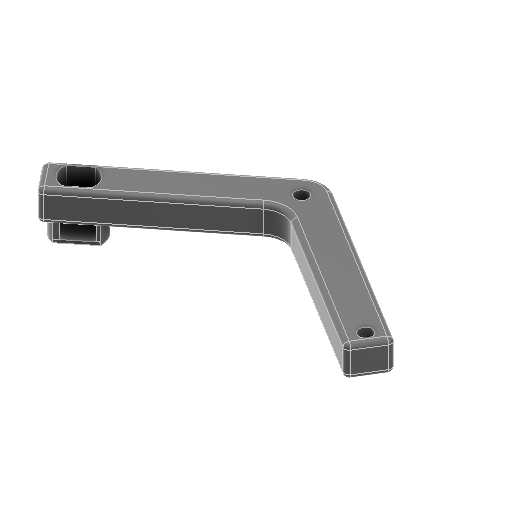
# Autodesk Inventor part: bogie
Saved by Autodesk Inventor 2025 (Build 290162010, 162A)
## iProperties
Created: 2024-08-06
Part Number: bogie
Material: Generic
Document SubType Name: Modeling
Designer: Pauline Simonnet
Density: 1 g/cm^3
Appearance: Smooth - Black
Author: Pauline Simonnet
Autodesk Inventor part; units mm, degrees
ref_plane "YZ Plane" through (0, 0, 0) normal (1, 0, 0) x (0, 1, 0)
ref_plane "XZ Plane" through (0, 0, 0) normal (0, 1, 0) x (-1, 0, 0)
ref_plane "XY Plane" through (0, 0, 0) normal (0, 0, 1) x (1, 0, 0)
sketch "Sketch1" plane through (0, 0, 0) normal (0, 1, 0) x (-1, 0, 0)
  line L0 (-464.4468, -188.2824) -> (-373.9516, -116.1994)
  line L1 (-373.9516, -116.1994) -> (-464.4468, -188.2824)
  line L2 (-464.4468, -188.2824) -> (-563.1339, -127.8985)
  line L3 (-563.1339, -127.8985) -> (-575.66, -148.3704)
  line L4 (-575.66, -148.3704) -> (-462.6384, -217.5251)
  line L5 (-373.9516, -116.1994) -> (-358.9986, -134.9719)
  line L6 (-358.9986, -134.9719) -> (-462.6384, -217.5251)
  line L7 (-462.6384, -217.5251) -> (-451.0106, -198.5213) construction
  line L8 (-462.6384, -217.5251) -> (-476.0378, -200.7031) construction
  circle A0 centre (-463.7684, -199.2538) radius 4.2
  circle A1 centre (-562.573, -142.3098) radius 4.3
  line L9 (-369.8895, -139.0445) -> (-380.7523, -147.6971)
  line L10 (-379.9517, -126.4122) -> (-390.8145, -135.0648)
  line L11 (-375.3209, -143.3708) -> (-385.3831, -130.7385) construction
  line L12 (-366.4751, -125.5857) -> (-380.352, -137.0546) construction
  arc A2 (-369.8895, -139.0445) -> (-379.9517, -126.4122) centre (-380.352, -137.0546) ccw
  arc A3 (-390.8145, -135.0648) -> (-380.7523, -147.6971) centre (-380.352, -137.0546) ccw
  point P0 (0, 0)
  dimension "d17" = 110
  dimension "d18" = 24
  dimension "d19" = 24
  dimension "d20" = 90
  dimension "d21" = 90
  dimension "d23" = 8.6
  dimension "d24" = 8.4
  dimension "d25" = 8
  dimension "d26" = 12
  dimension "d29" = 10.5
  dimension "d30" = 10.5
  dimension "d31" = 122
  dimension "d32" = 122
  dimension "d43" = 16.15
  dimension "d46" = 10.65
  dimension "d47" = 18
  constraints: 26 end point, 4 centre point, 4 midpoint, 4 point on circle, 1 coincident, 1 collinear, 1 perpendicular
  measures "d17" angle of L2 L0
  measures "d18" distance between parallel lines of L4 L2
  measures "d19" distance between parallel lines of L0 L6
  measures "d20" angle of L8 L6
  measures "d21" angle of L4 L7
  measures "d23" diameter of A1
  measures "d24" diameter of A0
  measures "d25" distance from line of L3 A1.centre
  measures "d26" distance from line of A1.centre L2
  measures "d29" distance from line of A0.centre L7
  measures "d30" distance from line of L8 A0.centre
  measures "d31" distance from line of L3 A0.centre
  measures "d32" distance from line of A0.centre L5
  measures "d43" distance between parallel lines of L10 L9
  measures "d46" radius of A3
  measures "d47" distance between parallel lines of L11 L5
extrude "Extrusion1" add sketch "Sketch1" along normal blind 20
fillet "Fillet1" radius 15 1 edges at (464.4468, 10, -188.2824)
fillet "Fillet2" radius 15 1 edges at (462.6384, 10, -217.5251)
fillet "Fillet3" radius 3 2 edges at (518.2699, 20, -155.3496) (415.0915, 20, -148.9689)
fillet "Fillet4" radius 3 3 edges at (462.8428, 20, -214.2198) (523.6288, 20, -180.2068) (406.7108, 20, -172.9766)
fillet "Fillet5" radius 3 3 edges at (462.8428, 0, -214.2198) (523.6288, 0, -180.2068) (406.7108, 0, -172.9766)
fillet "Fillet6" radius 3 2 edges at (518.2699, 0, -155.3496) (415.0915, 0, -148.9689)
fillet "Fillet7" radius 3 8 edges at (575.2014, 19.1213, -147.6209) (569.3969, 20, -138.1345) (563.5925, 19.1213, -128.6481) (563.1339, 10, -127.8985) (563.5925, 0.8787, -128.6481) (569.3969, 0, -138.1345) (575.2014, 0.8787, -147.6209) (575.66, 10, -148.3704)
fillet "Fillet8" radius 3 8 edges at (373.4042, 0.8787, -116.8867) (373.9516, 10, -116.1994) (373.4042, 19.1213, -116.8867) (366.4751, 20, -125.5857) (359.5461, 19.1213, -134.2846) (358.9986, 10, -134.9719) (359.5461, 0.8787, -134.2846) (366.4751, 0, -125.5857)
sketch "Sketch4" plane through (0, 0, 0) normal (0, -1, 0) x (1, 0, 0)
  arc A0 (379.9517, -126.4122) -> (369.8895, -139.0445) centre (380.352, -137.0546) ccw projected
  line L0 (368.3625, -139.1066) -> (381.7905, -149.8025)
  line L1 (369.8895, -139.0445) -> (380.7523, -147.6971) projected
  line L2 (365.9508, -139.7425) -> (380.5842, -151.3986)
  line L3 (394.6978, -137.0546) -> (377.3241, -122.7211)
  line L4 (454.3623, -184.0851) -> (374.4291, -120.4151) projected
  arc A1 (377.3241, -122.7211) -> (365.9508, -139.7425) centre (380.352, -137.0546) ccw
  arc A2 (380.5842, -151.3986) -> (394.6891, -136.553) centre (380.352, -137.0546) ccw
  arc A3 (380.0527, -124.8945) -> (368.3625, -139.1066) centre (380.352, -137.0546) ccw
  arc A4 (381.7905, -149.8025) -> (393.0533, -135.25) centre (380.352, -137.0546) ccw
  point P0 (0, 0)
  point P1 (379.9617, -124.8971)
  point P2 (393.1141, -135.748)
  dimension "d60" = 0
  dimension "d61" = 0
  dimension "d64" = 1
  dimension "d65" = 2
  constraints: 9 point on circle, 6 end point, 4 centre point, 4 point on line, 1 coincident, 1 parallel
  measures "d60" distance of A0.centre A3.centre
  measures "d61" distance of A0.centre A3.centre
  measures "d64" distance between parallel lines of L1 L0
  measures "d65" distance between parallel lines of L0 L2
extrude "Extrusion4" add sketch "Sketch4" along normal blind 10 contours L0 A4 L3 A2 L2 A1 A3
sketch "Sketch5" plane through (0, -10, 0) normal (0, -1, 0) x (1, 0, 0)
  arc A0 (383.8842, -150.9588) -> (394.6978, -137.0546) centre (380.352, -137.0546) ccw projected
  line L0 (394.6978, -137.0546) -> (377.413, -123.1311)
  arc A1 (380.5842, -151.3986) -> (394.6978, -137.0546) centre (380.352, -137.0546) ccw projected
  line L1 (380.5842, -151.3986) -> (365.9508, -139.7425)
  line L2 (365.9508, -139.7425) -> (380.5842, -151.3986) projected
  arc A2 (380.5842, -151.3986) -> (394.697, -136.8974) centre (380.352, -137.0546) ccw
  arc A3 (377.2325, -122.7407) -> (365.9508, -139.7425) centre (380.352, -137.0546) ccw
  line L3 (394.697, -136.8974) -> (377.2325, -122.7407)
  point P0 (0, 0)
  point P1 (377.5201, -122.8772)
  constraints: 8 end point, 4 point on circle, 2 centre point, 1 coincident
extrude "Extrusion5" add sketch "Sketch5" along normal blind 2
sketch "Sketch6" plane through (0, 0, 0) normal (0, -1, 0) x (1, 0, 0)
  circle A0 centre (463.7684, -199.2538) radius 11.425
  circle A1 centre (463.7684, -199.2538) radius 4.2 projected
  point P0 (0, 0)
  dimension "d70" = 0
  dimension "d71" = 0
  dimension "d72" = 22.85
  constraints: 1 centre point
  measures "d70" distance of A1.centre A0.centre
  measures "d71" distance of A1.centre A0.centre
  measures "d72" diameter of A0
extrude "Extrusion6" cut sketch "Sketch6" against normal blind 10
body "Solid1"
